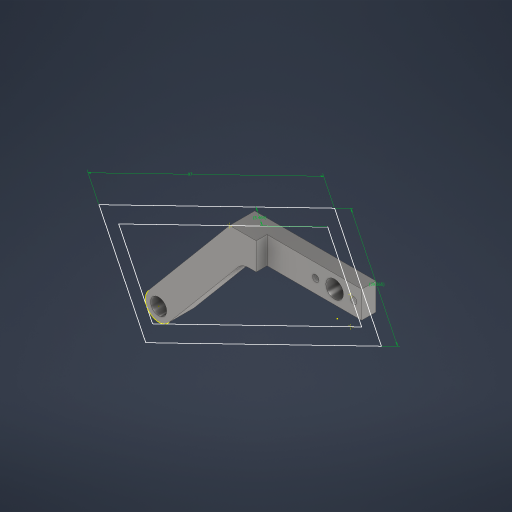
# Autodesk Inventor part: Servo_Strut_v2
Saved by Autodesk Inventor 2023 (Build 270158000, 158)
## iProperties
Created: 2023-02-25
Part Number: Servo_Strut_v2
Material: Steel, Carbon
Document SubType Name: Modeling
Designer: roota
Density: 7.85 g/cm^3
Appearance: Semi-Polished
Mass: 33.4264 g
Surface Area: 27.0753 cm^2
Volume: 4.25814 cm^3
Author: roota
Autodesk Inventor part; units mm, degrees
ref_plane "YZ Plane" through (0, 0, 0) normal (1, 0, 0) x (0, 1, 0)
ref_plane "XZ Plane" through (0, 0, 0) normal (0, 1, 0) x (-1, 0, 0)
ref_plane "XY Plane" through (0, 0, 0) normal (0, 0, 1) x (1, 0, 0)
sketch "Sketch1" plane through (0, 0, 0) normal (0, 0, 1) x (1, 0, 0)
  line L0 (0, 0) -> (-35.2056, 0)
  line L1 (-35.2056, 0) -> (-65.5234, -36.1314)
  line L2 (-65.5234, -36.1314) -> (-73.1839, -29.7035)
  line L3 (-73.1839, -29.7035) -> (-39.8687, 10)
  line L4 (-39.8687, 10) -> (0, 10)
  line L5 (0, 10) -> (0, 0)
  circle A0 centre (-66.1397, -29.0872) radius 3
  circle A1 centre (-5, 5) radius 3.25
  line L6 (0, 5) -> (-37.5371, 5) construction
  line L7 (-37.5371, 5) -> (-69.3536, -32.9174) construction
  line L8 (0, 0) -> (-65.5234, -36.1314) construction
  line L9 (0, 10) -> (5, 10)
  line L10 (5, 10) -> (5, 0)
  line L11 (5, 0) -> (0, 0)
  line L12 (0, 0) -> (0, 10)
  dimension "d0" = 10
  dimension "d1" = 6
  dimension "d2" = 6.5
  dimension "d3" = 5
  dimension "d4" = 5
  dimension "d5" = 70
  dimension "d26" = 50
  dimension "d28" = 17
  dimension "d37" = 5
  constraints: 26 end point, 4 parallel, 4 perpendicular, 3 horizontal, 2 centre point, 2 midpoint, 2 point on line, 1 equal length
  measures "d0" distance of L4.end L0.start
  measures "d1" diameter of A0
  measures "d2" diameter of A1
  measures "d3" distance from line of L5 A1.centre
  measures "d4" distance from line of L2 A0.centre
  measures "d5" distance of A1.centre A0.centre
  measures "d26" angle of L7 L0
  measures "d28" distance from line of L0.end L8
  measures "d37" distance between parallel lines of L5 L10
extrude "Extrusion1" add sketch "Sketch1" along normal blind 9.3
fillet "Fillet1" radius 5 3 edges at (-73.1839, -29.7035, 4.65) (-65.5234, -36.1314, 4.65) (-35.2056, 0, 4.65)
sketch "Sketch5" plane through (0, 0, 0) normal (0, 0, -1) x (-1, 0, 0)
  circle A0 centre (5, 5) radius 3.25 projected
  point P0 (0, 0)
  point P1 (12, 5)
  point P2 (-2, 5)
  dimension "d29" = 7
  dimension "d38" = 7
  constraints: 2 horizontal alignment
  measures "d29" distance of A0.centre point (12, 5)
  measures "d38" distance of A0.centre point (-2, 5)
hole "Hole1" at (-12, 5, 0) at (2, 5, 0) direction (0, 0, 1) diameter 2.459 end through all thread size "M3x0.5" class "6H" standard "ISO Metric profile"
sketch "Sketch4" plane through (0, 0, 9.3) normal (0, 0, 1) x (1, 0, 0)
  line L0 (0, 0) -> (-30, 0)
  line L1 (-30, 0) -> (-30, 10)
  line L2 (-30, 10) -> (0, 10)
  line L3 (0, 10) -> (0, 0)
  line L4 (0, 10) -> (5, 10)
  line L5 (5, 10) -> (5, 0)
  line L6 (5, 0) -> (0, 0)
  line L7 (0, 0) -> (0, 10)
  dimension "d20" = 30
  constraints: 16 end point, 4 parallel, 2 coincident, 2 horizontal, 2 perpendicular
  measures "d20" distance of L1.end L2.end
extrude "Extrusion4" cut sketch "Sketch4" against normal blind 4
sketch "Sketch6" plane through (0, 0, 9.3) normal (0, 0, 1) x (1, 0, 0)
  line L0 (-3.6029, 27.6633) -> (-80.9851, -10.0258)
  line L1 (-80.9851, -10.0258) -> (-68.4455, -35.7718)
  line L2 (-68.4455, -35.7718) -> (8.9367, 1.9174)
  line L3 (8.9367, 1.9174) -> (-3.6029, 27.6633)
  arc A0 (-69.9699, -25.8733) -> (-62.3095, -32.3011) centre (-66.1397, -29.0872) ccw projected
  line L4 (-88.2897, -7.5062) -> (-1.0833, 34.9679)
  line L5 (-1.0833, 34.9679) -> (16.2412, -0.6023)
  line L6 (16.2412, -0.6023) -> (-70.9652, -43.0763)
  line L7 (-70.9652, -43.0763) -> (-88.2897, -7.5062)
  point P0 (0, 0)
  point P1 (5, 10)
  point P2 (-39.8687, 10)
  point P3 (5, 0)
  dimension "d39" = 97
  dimension "d40" = 39.5648
  dimension "d41" = 5.4638
  constraints: 16 end point, 4 parallel, 3 point on line, 2 perpendicular, 2 tangent, 3 other
  measures "d39" distance of L4.start L4.end
  measures "d40" distance of L4.end L5.end
  measures "d41" distance between parallel lines of L4 L0
equation "\"d3\" = 0.5 * d0"
equation "\"d4\" = 0.5 * d0"
equation "\"d38\" = d29"
body "Solid1"
